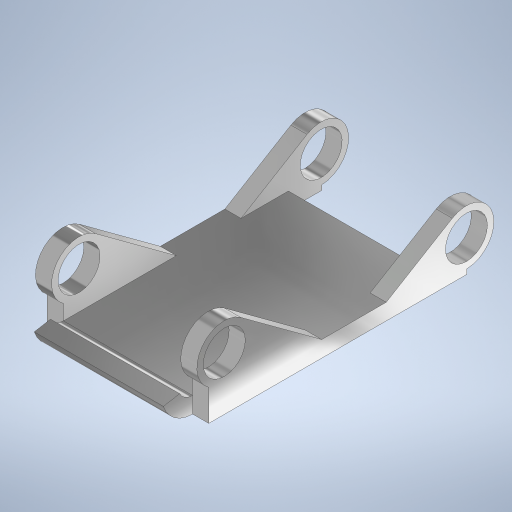
# Autodesk Inventor part: D26 linkage
Saved by Autodesk Inventor 2024 (Build 280153000, 153)
## iProperties
Perskaiciuoti: 1
Created: 2006-11-26
Part Number: D26 linkage
Document SubType Name: Modeling
Designer: G.K.
Description: Linkage
Authority: Design by UAB Čeli APS
Material: Steel
Mass: 1.54209 g
Surface Area: 5.06964 cm^2
Volume: 0.196444 cm^3
Density: 7.85 g/cm^3
Appearance: Chrome - Polished
Pavadinimas: Aselė
Šifras: L-90.00 002
Mase: 0.00154209
Autodesk Inventor part; units mm, degrees
ref_plane "YZ Plane" through (0, 0, 0) normal (1, 0, 0) x (0, 1, 0)
ref_plane "XZ Plane" through (0, 0, 0) normal (0, 1, 0) x (-1, 0, 0)
ref_plane "XY Plane" through (0, 0, 0) normal (0, 0, 1) x (1, 0, 0)
sketch "Sketch2" plane through (0, 0, 0) normal (1, 0, 0) x (0, 1, 0)
  line L0 (0, 7.6453) -> (0, -1.2742) projected
  line L1 (7, 0.6675) -> (7, 0.9678)
  arc A0 (-7.0268, 5.3689) -> (-9, 2.6006) centre (-8.0348, 4) ccw
  line L2 (-9, 2.6006) -> (-9, 0.6675)
  line L3 (2, 1.6675) -> (6.0897, 4.1247)
  arc A1 (7, 0.9678) -> (6.0897, 4.1247) centre (6.9652, 2.6675) ccw
  circle A2 centre (6.9652, 2.6675) radius 1.3
  circle A3 centre (-8.0348, 4) radius 1.3
  line L4 (2, 1.6675) -> (-2, 1.6675)
  circle A4 centre (-8.0348, 4) radius 1.3
  line L5 (7, 0.6675) -> (-9, 0.6675)
  line L6 (-2, 1.6675) -> (-7.0268, 5.3689)
  point P0 (0, 1.6675)
  point P1 (0, 0)
  dimension "d6" = 1.7
  dimension "d17" = 2.6
  dimension "d61" = 2.6
  dimension "d62" = 1.7
  dimension "d76" = 15
  dimension "d77" = 0.6675
  dimension "d79" = 2
  dimension "d80" = 4
  dimension "d81" = 1
  dimension "d84" = 16
  dimension "d85" = 9
  constraints: 12 end point, 5 centre point, 4 point on circle, 3 coincident, 3 perpendicular, 2 tangent, 1 equal radius, 1 midpoint, 1 parallel, 1 point on line, 2 other
  measures "d6" radius of A1
  measures "d17" diameter of A2
  measures "d61" diameter of A4
  measures "d62" radius of A0
  measures "d76" horizontal distance of A0.centre A1.centre
  measures "d77" distance from line of point (0, 0) L5
  measures "d79" distance from line of A1.centre L5
  measures "d80" distance of L3.start L4.end
  measures "d81" distance between parallel lines of L5 L4
  measures "d84" distance between parallel lines of L1 L2
  measures "d85" distance between parallel lines of L0 L2
extrude "Extrusion1" add sketch "Sketch2" along normal mid plane 10
sketch "Sketch4" plane through (0, 0, 0) normal (1, 0, 0) x (0, 1, 0)
  line L0 (-10.8077, 1.9824) -> (-9.8024, 2.1597)
  line L1 (7, 0.6675) -> (-9, 0.6675) projected
  arc A0 (-10.8077, 1.9824) -> (-9, 0.6675) centre (-9, 2.5675) ccw
  arc A1 (-9.8024, 2.1597) -> (-9, 1.6674) centre (-9, 2.5675) ccw
  line L2 (-9, 0.6675) -> (-9, 2.6006) projected
  dimension "d66" = 0.9001
  dimension "d67" = 1.9
  dimension "d68" = 80
  dimension "d69" = 0.8024
  constraints: 4 point on circle, 3 end point, 2 centre point, 1 coincident, 1 point on line, 1 tangent
  measures "d66" radius of A1
  measures "d67" radius of A0
  measures "d68" angle of L0 L2
  measures "d69" distance from line of L2 L0.end
extrude "Extrusion3" add sketch "Sketch4" along normal mid plane 8
sketch "Sketch5" plane through (-5, 2, 1.6675) normal (0, 0, 1) x (1, 0, 0)
  line L0 (1, 6.6652) -> (9, 6.6652)
  line L1 (9, 6.6652) -> (9, -11)
  line L2 (1, -11) -> (1, 6.6652)
  line L3 (1, -11.8024) -> (1, -12.8077) projected
  line L4 (9, -12.8077) -> (9, -11.8024) projected
  line L5 (0, 6.6652) -> (10, 6.6652) projected
  line L6 (0, -4) -> (10, -4) projected
  line L7 (1, -11) -> (9, -11)
  line L8 (0, -11) -> (1, -11) projected
  point P0 (5, -2)
  constraints: 8 end point, 4 collinear, 2 parallel, 1 horizontal, 1 perpendicular
extrude "Extrusion4" cut sketch "Sketch5" along normal through all
sketch "Sketch6" plane through (-5, -2, 1.6675) normal (0, 0, 1) x (1, 0, 0)
  line L0 (9, 8.1346) -> (9, 4) projected
  line L1 (1, 8.1346) -> (9, 8.1346) projected
  line L2 (1, 4) -> (1, 8.1346) projected
  line L3 (9, 6.9346) -> (1, 6.9346)
  line L4 (1, 6.9346) -> (1, 11.9346)
  line L5 (1, 11.9346) -> (9, 11.9346)
  line L6 (9, 11.9346) -> (9, 6.9346)
  point P0 (5, 2)
  dimension "d72" = 1.2
  dimension "d73" = 5
  constraints: 8 end point, 2 parallel, 1 collinear, 1 horizontal, 1 perpendicular, 1 point on line
  measures "d72" distance between parallel lines of L1 L3
  measures "d73" distance between parallel lines of L3 L5
extrude "Extrusion5" cut sketch "Sketch6" against normal through all
delete faces "Delete Face1" heal yes whole lump no faces at (1.3333, -9, 5.047) (1.3333, -9, 2.7768)
body "Solid1"
